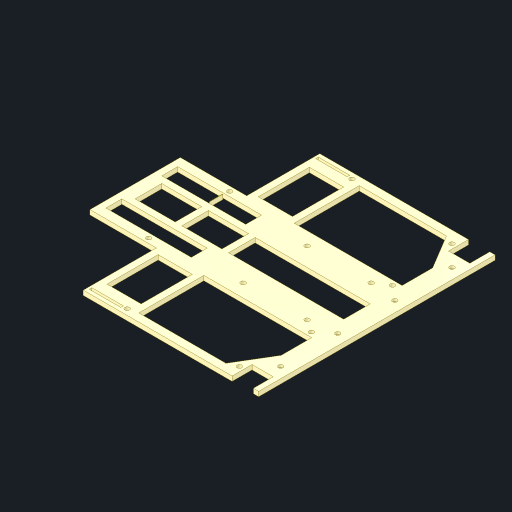
# Autodesk Inventor part: base
Saved by Autodesk Inventor 2023 (Build 270158000, 158)
## iProperties
Created: 2024-04-29
Part Number: base
Material: Nylon 6/6
Document SubType Name: Modeling
Designer: szymo
Density: 1.13 g/cm^3
Appearance: Nylon 6
Mass: 48.7008 g
Surface Area: 329.425 cm^2
Volume: 43.0981 cm^3
Author: szymo
Autodesk Inventor part; units mm, degrees
ref_plane "YZ Plane" through (0, 0, 0) normal (1, 0, 0) x (0, 1, 0)
ref_plane "XZ Plane" through (0, 0, 0) normal (0, 1, 0) x (-1, 0, 0)
ref_plane "XY Plane" through (0, 0, 0) normal (0, 0, 1) x (1, 0, 0)
sketch "Sketch1" plane through (0, 0, 0) normal (0, 1, 0) x (-1, 0, 0)
  line L0 (99, 89) -> (-99, 89)
  line L1 (-99, 89) -> (-99, -89)
  line L2 (-99, -89) -> (99, -89)
  line L3 (99, -89) -> (99, 89)
  line L4 (99, 89) -> (-99, -89) construction
  line L5 (-99, 89) -> (99, -89) construction
  line L6 (-99, 89) -> (-85, 89)
  line L7 (-85, 89) -> (-85, -89)
  line L8 (-85, -89) -> (-99, -89)
  line L9 (-99, -89) -> (-99, 89)
  line L10 (99, 89) -> (97, 89)
  line L11 (97, 89) -> (97, -89)
  line L12 (97, -89) -> (99, -89)
  line L13 (99, -89) -> (99, 89)
  line L14 (97, 33) -> (97, 35)
  line L15 (97, -33) -> (97, -35)
  line L16 (97, 32.8) -> (97, 35)
  line L17 (97, -32.8) -> (97, -35)
  line L18 (97, 89) -> (47, 89)
  line L19 (47, 89) -> (47, 34)
  line L20 (47, 34) -> (97, 34)
  line L21 (97, 34) -> (97, 89)
  line L22 (97, -89) -> (47, -89)
  line L23 (47, -89) -> (47, -34)
  line L24 (47, -34) -> (97, -34)
  line L25 (97, -34) -> (97, -89)
  line L26 (66.5, 33) -> (77.5, 33) projected
  line L27 (77.5, -33) -> (66.5, -33) projected
  line L28 (-81, 74) -> (-81, 89) projected
  line L29 (-81, 31) -> (-81, 55) projected
  line L30 (-81, -12) -> (-81, 12) projected
  line L31 (-81, -55) -> (-81, -31) projected
  line L32 (-81, -89) -> (-81, -74) projected
  arc A0 (-81, 74) -> (-79, 72) centre (-79, 74) ccw projected
  line L33 (-70, 72) -> (-79, 72) projected
  line L34 (-70, 57) -> (-70, 72) projected
  line L35 (-79, 57) -> (-70, 57) projected
  arc A1 (-79, 57) -> (-81, 55) centre (-79, 55) ccw projected
  arc A2 (-81, 31) -> (-79, 29) centre (-79, 31) ccw projected
  line L36 (-70, 29) -> (-79, 29) projected
  line L37 (-70, 14) -> (-70, 29) projected
  line L38 (-79, 14) -> (-70, 14) projected
  arc A3 (-79, 14) -> (-81, 12) centre (-79, 12) ccw projected
  arc A4 (-81, -12) -> (-79, -14) centre (-79, -12) ccw projected
  line L39 (-70, -14) -> (-79, -14) projected
  line L40 (-70, -29) -> (-70, -14) projected
  line L41 (-79, -29) -> (-70, -29) projected
  arc A5 (-79, -29) -> (-81, -31) centre (-79, -31) ccw projected
  arc A6 (-81, -55) -> (-79, -57) centre (-79, -55) ccw projected
  line L42 (-70, -57) -> (-79, -57) projected
  line L43 (-70, -72) -> (-70, -57) projected
  line L44 (-79, -72) -> (-70, -72) projected
  arc A7 (-79, -72) -> (-81, -74) centre (-79, -74) ccw projected
  circle A8 centre (-77, -64.5) radius 1.2295 projected
  circle A9 centre (-77, -21.5) radius 1.2295 projected
  circle A10 centre (-77, 21.5) radius 1.2295 projected
  circle A11 centre (-77, 64.5) radius 1.2295 projected
  line L45 (-65, 89) -> (-79, 89)
  line L46 (-79, 89) -> (-79, 75)
  line L47 (-79, 75) -> (-65, 75)
  line L48 (-65, 75) -> (-65, 89)
  line L49 (-65, 89) -> (-81, 89)
  line L50 (-81, 89) -> (-81, 74)
  line L51 (-81, 74) -> (-65, 74)
  line L52 (-65, 74) -> (-65, 89)
  line L53 (-99, 0) -> (97, 0)
  line L54 (0, 0) -> (-99, 0) construction
  line L55 (-65, -89) -> (-79, -89)
  line L56 (-79, -89) -> (-79, -75)
  line L57 (-79, -75) -> (-65, -75)
  line L58 (-65, -75) -> (-65, -89)
  line L59 (-65, -89) -> (-81, -89)
  line L60 (-81, -89) -> (-81, -74)
  line L61 (-81, -74) -> (-65, -74)
  line L62 (-65, -74) -> (-65, -89)
  point P0 (47, 89)
  point P1 (47, -89)
  point P2 (97, 34)
  point P3 (-81, -89)
  point P4 (-79, -74)
  dimension "d0" = 198
  dimension "d1" = 178
  dimension "d2" = 14
  dimension "d3" = 2
  dimension "d16" = 50
  dimension "d17" = 55
  dimension "d18" = 50
  dimension "d19" = 55
  dimension "d20" = 1
  dimension "d21" = 1
  dimension "d22" = 14
  dimension "d23" = 14
  dimension "d24" = 2
  dimension "d25" = 1
  dimension "d26" = 2
  constraints: 88 end point, 14 parallel, 10 symmetric about line, 8 perpendicular, 8 point on line, 7 horizontal, 4 midpoint, 2 collinear
  measures "d0" distance of L2.end L1.end
  measures "d1" distance of L1.end L0.end
  measures "d2" distance of L7.end L8.end
  measures "d3" distance of L12.end L11.end
  measures "d16" distance of L20.end L19.end
  measures "d17" distance of L19.end L18.end
  measures "d18" distance of L23.end L24.end
  measures "d19" distance of L22.end L23.end
  measures "d20" distance between parallel lines of L20 L26
  measures "d21" distance between parallel lines of L27 L24
  measures "d22" distance of L47.end L46.end
  measures "d23" distance of L46.end L45.end
  measures "d24" distance between parallel lines of L28 L46
  measures "d25" distance between parallel lines of L47 L51
  measures "d26" distance between parallel lines of L33 L51
extrude "Extrusion1" add sketch "Sketch1" along normal blind 3.5 contours L19 L20 L11 L53 L30 A3 L38 L37 L36 A2 L29 A1 L35 L34 L33 A0 L51 L52 L48 L0 | L2 L58 L62 L61 A7 L44 L43 L42 A6 L31 A5 L41 L40 L39 A4 L30 L53 L11 L24 L23 | L28 A0 L33 L34 L35 A1 L29 A2 L36 L37 L38 A3 L30 L53 L7 L0 | L2 L7 L53 L30 A4 L39 L40 L41 A5 L31 A6 L42 L43 L44 A7 L32 | A8 | A9 | A10 | A11
sketch "Sketch3" plane through (0, 0, 0) normal (0, -1, 0) x (1, 0, 0)
  line L0 (65, -74) -> (65, -89) projected
  line L1 (81, -74) -> (65, -74) projected
  line L2 (81, -89) -> (81, -74) projected
  line L3 (85, -89) -> (81, -89) projected
  line L4 (85, 89) -> (85, -89) projected
  line L5 (81, 89) -> (85, 89) projected
  line L6 (81, 74) -> (81, 89) projected
  line L7 (65, 74) -> (81, 74) projected
  line L8 (65, 89) -> (65, 74) projected
  line L9 (-47, 89) -> (65, 89) projected
  line L10 (-47, 34) -> (-47, 89) projected
  line L11 (-97, 34) -> (-47, 34) projected
  line L12 (-97, -34) -> (-97, 34) projected
  line L13 (-47, -34) -> (-97, -34) projected
  line L14 (-47, -89) -> (-47, -34) projected
  line L15 (65, -89) -> (-47, -89) projected
  circle A0 centre (70, 80) radius 1.75 projected
  line L16 (-21.635, 86.2) -> (-21.635, 84.2) projected
  line L17 (-21.635, 84.2) -> (-45.325, 84.2) projected
  line L18 (-45.325, 84.2) -> (-45.325, 86.2) projected
  line L19 (-45.325, 86.2) -> (-21.635, 86.2) projected
  line L20 (73, 77) -> (73, 89) projected
  line L21 (-47, 89) -> (73, 89) projected
  line L22 (-47, 89) -> (-47, 76.2) projected
  line L23 (-14.925, 76.2) -> (-47, 76.2) projected
  line L24 (-14.925, 83) -> (-14.925, 76.2) projected
  line L25 (58, 83) -> (-14.925, 83) projected
  line L26 (58, 77) -> (58, 83) projected
  line L27 (73, 77) -> (58, 77) projected
  circle A1 centre (-18.3706, 84.6) radius 1.8 projected
  circle A2 centre (61.5, 80) radius 1.8 projected
  circle A3 centre (70, -83) radius 1.75 projected
  line L28 (-21.635, -86.2) -> (-21.635, -84.2) projected
  line L29 (-45.325, -86.2) -> (-21.635, -86.2) projected
  line L30 (-45.325, -84.2) -> (-45.325, -86.2) projected
  line L31 (-21.635, -84.2) -> (-45.325, -84.2) projected
  line L32 (73, -77) -> (73, -89) projected
  line L33 (73, -77) -> (58, -77) projected
  line L34 (58, -77) -> (58, -83) projected
  line L35 (58, -83) -> (-14.925, -83) projected
  line L36 (-14.925, -83) -> (-14.925, -76.2) projected
  line L37 (-14.925, -76.2) -> (-47, -76.2) projected
  line L38 (-47, -89) -> (-47, -76.2) projected
  line L39 (-47, -89) -> (73, -89) projected
  circle A4 centre (-18.3706, -84.6) radius 1.8 projected
  circle A5 centre (61.5, -80) radius 1.8 projected
  line L40 (-16.25, -37.7) -> (-47, -37.7) projected
  line L41 (-16.25, -37.7) -> (-16.25, -34.2) projected
  line L42 (-16.25, -34.2) -> (-47, -34.2) projected
  line L43 (-47, -37.7) -> (-47, -34.2) projected
  circle A6 centre (66.25, -30.5) radius 1.8 projected
  circle A7 centre (-56.325, -30.5) radius 1.8 projected
  line L44 (69.5, -34) -> (69.5, -27) projected
  line L45 (69.5, -27) -> (-97, -27) projected
  line L46 (-97, -27) -> (-97, -34) projected
  line L47 (-97, -34) -> (-94, -34) projected
  line L48 (-94, -34) -> (41.0514, -34) projected
  line L49 (41.0514, -34) -> (41.0514, -45) projected
  line L50 (41.0514, -45) -> (45.7494, -45) projected
  line L51 (45.7494, -45) -> (45.7494, -34.8203) projected
  line L52 (45.7494, -45) -> (59.075, -45) projected
  line L53 (59.075, -34) -> (59.075, -45) projected
  line L54 (59.075, -34) -> (69.5, -34) projected
  line L55 (-16.65, -10) -> (-16.65, -27) projected
  line L56 (-16.65, -10) -> (-97, -10) projected
  line L57 (-97, -15) -> (-97, -10) projected
  line L58 (-97, -15) -> (-17.65, -15) projected
  line L59 (-17.65, -15) -> (-17.65, -27) projected
  line L60 (-16.65, -27) -> (-17.65, -27) projected
  line L61 (-16.65, 10) -> (-16.65, 27) projected
  line L62 (-16.65, 27) -> (-17.65, 27) projected
  line L63 (-17.65, 15) -> (-17.65, 27) projected
  line L64 (-97, 15) -> (-17.65, 15) projected
  line L65 (-97, 15) -> (-97, 10) projected
  line L66 (-16.65, 10) -> (-97, 10) projected
  line L67 (-16.25, 37.7) -> (-47, 37.7) projected
  line L68 (-47, 37.7) -> (-47, 34.2) projected
  line L69 (-16.25, 34.2) -> (-47, 34.2) projected
  line L70 (-16.25, 37.7) -> (-16.25, 34.2) projected
  circle A8 centre (66.25, 30.5) radius 1.8 projected
  circle A9 centre (-56.325, 30.5) radius 1.8 projected
  line L71 (69.5, 34) -> (69.5, 27) projected
  line L72 (59.075, 34) -> (69.5, 34) projected
  line L73 (59.075, 34) -> (59.075, 45) projected
  line L74 (45.7494, 45) -> (59.075, 45) projected
  line L75 (45.7494, 45) -> (45.7494, 34.8203) projected
  line L76 (41.0514, 45) -> (45.7494, 45) projected
  line L77 (41.0514, 34) -> (41.0514, 45) projected
  line L78 (-94, 34) -> (41.0514, 34) projected
  line L79 (-97, 34) -> (-94, 34) projected
  line L80 (-97, 27) -> (-97, 34) projected
  line L81 (69.5, 27) -> (-97, 27) projected
  circle A10 centre (77, 21.5) radius 1.2295 projected
  circle A11 centre (77, -64.5) radius 1.2295 projected
  circle A12 centre (77, -21.5) radius 1.2295 projected
  circle A13 centre (77, 64.5) radius 1.2295 projected
  line L82 (70, -72) -> (79, -72) projected
  arc A14 (81, -74) -> (79, -72) centre (79, -74) ccw projected
  line L83 (81, -74) -> (81, -89) projected
  line L84 (81, -89) -> (85, -89) projected
  line L85 (85, -89) -> (85, 89) projected
  line L86 (81, 89) -> (85, 89) projected
  line L87 (81, 89) -> (81, 74) projected
  arc A15 (79, 72) -> (81, 74) centre (79, 74) ccw projected
  line L88 (79, 72) -> (70, 72) projected
  line L89 (70, 57) -> (70, 72) projected
  line L90 (70, 57) -> (79, 57) projected
  arc A16 (81, 55) -> (79, 57) centre (79, 55) ccw projected
  line L91 (81, 55) -> (81, 31) projected
  arc A17 (79, 29) -> (81, 31) centre (79, 31) ccw projected
  line L92 (79, 29) -> (70, 29) projected
  line L93 (70, 14) -> (70, 29) projected
  line L94 (70, 14) -> (79, 14) projected
  arc A18 (81, 12) -> (79, 14) centre (79, 12) ccw projected
  line L95 (81, 12) -> (81, -12) projected
  arc A19 (79, -14) -> (81, -12) centre (79, -12) ccw projected
  line L96 (79, -14) -> (70, -14) projected
  line L97 (70, -29) -> (70, -14) projected
  line L98 (70, -29) -> (79, -29) projected
  arc A20 (81, -31) -> (79, -29) centre (79, -31) ccw projected
  line L99 (81, -31) -> (81, -55) projected
  arc A21 (79, -57) -> (81, -55) centre (79, -55) ccw projected
  line L100 (79, -57) -> (70, -57) projected
  line L101 (70, -72) -> (70, -57) projected
  line L102 (85, 89) -> (70, 89)
  line L103 (70, 89) -> (70, -89)
  line L104 (65, -89) -> (85, -89)
  line L105 (85, -89) -> (85, 89)
  line L106 (85, 34) -> (-97, 34)
  line L107 (-97, 34) -> (-97, 10)
  line L108 (-97, 10) -> (85, 10)
  line L109 (85, 10) -> (85, 34)
  line L110 (-97, -10) -> (85, -10)
  line L111 (85, -10) -> (85, -34)
  line L112 (85, -34) -> (-97, -34)
  line L113 (-97, -34) -> (-97, -10)
  line L114 (-47, 34) -> (-47, 34.2)
  line L115 (-47, 34.2) -> (-97, 34)
  line L116 (-97, -34) -> (-47, -34.2)
  line L117 (-47, -34.2) -> (-47, -34)
  line L118 (70, 89) -> (58, 89)
  line L119 (58, 89) -> (58, 77)
  line L120 (58, 77) -> (70, 77)
  line L121 (70, 77) -> (70, 89)
  line L122 (58, 89) -> (-14.925, 89)
  line L123 (-14.925, 89) -> (-14.925, 83)
  line L124 (-14.925, 83) -> (58, 83)
  line L125 (58, 83) -> (58, 89)
  line L126 (-14.925, 89) -> (-47, 89)
  line L127 (-47, 89) -> (-47, 76.2)
  line L128 (-47, 76.2) -> (-14.925, 76.2)
  line L129 (-14.925, 76.2) -> (-14.925, 89)
  line L130 (65, -77) -> (58, -77)
  line L131 (58, -77) -> (58, -89)
  line L132 (58, -89) -> (70, -89)
  line L133 (70, -89) -> (70, -77)
  line L134 (58, -89) -> (-14.925, -89)
  line L135 (-14.925, -89) -> (-14.925, -83)
  line L136 (-14.925, -83) -> (58, -83)
  line L137 (58, -83) -> (58, -89)
  line L138 (-14.925, -89) -> (-47, -89)
  line L139 (-47, -89) -> (-47, -76.2)
  line L140 (-47, -76.2) -> (-14.925, -76.2)
  line L141 (-14.925, -76.2) -> (-14.925, -89)
  line L142 (-47, -76.2) -> (-42, -76.2)
  line L143 (-42, -76.2) -> (-42, -34)
  line L144 (-42, -34) -> (-47, -34)
  line L145 (-47, -34) -> (-47, -76.2)
  line L146 (-47, 76.2) -> (-42, 76.2)
  line L147 (-42, 76.2) -> (-42, 34)
  line L148 (-42, 34) -> (-47, 34)
  line L149 (-47, 34) -> (-47, 76.2)
  line L150 (-16.25, 34.2) -> (-11.25, 34.2)
  line L151 (-11.25, 34.2) -> (-11.25, 83)
  line L152 (-11.25, 83) -> (-16.25, 83)
  line L153 (-16.25, 83) -> (-16.25, 34.2)
  line L154 (-16.25, -34.2) -> (-11.25, -34.2)
  line L155 (-11.25, -34.2) -> (-11.25, -83)
  line L156 (-11.25, -83) -> (-16.25, -83)
  line L157 (-16.25, -83) -> (-16.25, -34.2)
  line L158 (-16.65, 10) -> (-21.65, 10)
  line L159 (-21.65, 10) -> (-21.65, -10)
  line L160 (-21.65, -10) -> (-16.65, -10)
  line L161 (-16.65, -10) -> (-16.65, 10)
  line L162 (-97, 10) -> (-87, 10)
  line L163 (-87, 10) -> (-87, -10)
  line L164 (-87, -10) -> (-97, -10)
  line L165 (-97, -10) -> (-97, 10)
  line L166 (-51.825, 10) -> (-56.825, 10)
  line L167 (-56.825, 10) -> (-56.825, -10)
  line L168 (-56.825, -10) -> (-51.825, -10)
  line L169 (-51.825, -10) -> (-51.825, 10)
  line L170 (-16.25, 34.2) -> (-16.25, 34)
  line L171 (-11.25, 34.2) -> (-11.25, 34)
  line L172 (-11.25, -34.2) -> (-11.25, -34)
  line L173 (-16.25, -34.2) -> (-16.25, -34)
  line L174 (70, 57) -> (54.4, 83)
  line L175 (70, -57) -> (54.4, -83)
  line L176 (-34.0117, 16) -> (-34.0117, 26)
  line L177 (-34.0117, 26) -> (-32.704, 26)
  line L178 (-32.704, 26) -> (-32.704, 16)
  line L179 (-32.704, 16) -> (-34.0117, 16)
  line L180 (-35.6343, 26) -> (-35.6343, 16)
  line L181 (-35.6343, 16) -> (-50.4468, 16)
  line L182 (-50.4468, 16) -> (-50.4468, 26)
  line L183 (-50.4468, 26) -> (-35.6343, 26)
  line L184 (-66.4245, 19) -> (-72.4408, 19)
  line L185 (-72.4408, 19) -> (-72.4408, 23)
  line L186 (-72.4408, 23) -> (-66.4245, 23)
  line L187 (-66.4245, 23) -> (-66.4245, 19)
  line L188 (-82.583, 26) -> (-82.583, 23)
  line L189 (-82.583, 23) -> (-80.9671, 23)
  line L190 (-80.9671, 23) -> (-80.9671, 19)
  line L191 (-80.9671, 19) -> (-82.583, 19)
  line L192 (-82.583, 19) -> (-82.583, 16)
  line L193 (-82.583, 16) -> (-86.007, 16)
  spline S0 degree 3 poles (-86.007, 16) (-86.007, 17.6667) (-86.007, 19.3333) (-86.007, 22.6667) (-86.007, 24.3333) (-86.007, 26) knots -1 -1 -1 -1 -0.5 -0.5 0 0 0 0
  line L194 (-86.007, 26) -> (-82.583, 26)
  line L195 (-61.417, 23) -> (-61.417, 26)
  line L196 (-61.417, 26) -> (-57.3554, 26)
  spline S1 degree 3 poles (-57.3554, 26) (-57.3554, 24.3333) (-57.3554, 22.6667) (-57.3554, 19.3333) (-57.3554, 17.6667) (-57.3554, 16) knots -1 -1 -1 -1 -0.5 -0.5 0 0 0 0
  line L197 (-57.3554, 16) -> (-61.417, 16)
  line L198 (-61.417, 16) -> (-61.417, 19)
  line L199 (-61.417, 19) -> (-62.6269, 19)
  line L200 (-62.6269, 19) -> (-62.6269, 23)
  line L201 (-62.6269, 23) -> (-61.417, 23)
  line L202 (-57.2691, 26) -> (-57.2691, 16)
  line L203 (-86.7309, 16) -> (-86.7309, 26)
  line L204 (-49.6101, -16) -> (-49.6101, -26)
  line L205 (-49.6101, -26) -> (-51.9631, -26)
  line L206 (-51.9631, -26) -> (-51.9631, -16)
  line L207 (-51.9631, -16) -> (-49.6101, -16)
  line L208 (-33.7735, -16) -> (-33.7735, -26)
  line L209 (-33.7735, -26) -> (-49.1385, -26)
  line L210 (-49.1385, -26) -> (-49.1385, -16)
  line L211 (-49.1385, -16) -> (-33.7735, -16)
  line L212 (-61.417, -26) -> (-61.417, -23)
  line L213 (-61.417, -23) -> (-69.2128, -23)
  line L214 (-69.2128, -23) -> (-69.2128, -19)
  line L215 (-69.2128, -19) -> (-61.417, -19)
  line L216 (-61.417, -19) -> (-61.417, -16)
  line L217 (-61.417, -16) -> (-57.0283, -16)
  spline S2 degree 3 poles (-57.0283, -16) (-57.0283, -17.6667) (-57.0283, -19.3333) (-57.0283, -22.6667) (-57.0283, -24.3333) (-57.0283, -26) knots -1 -1 -1 -1 -0.5 -0.5 0 0 0 0
  line L218 (-57.0283, -26) -> (-61.417, -26)
  line L219 (-82.583, -23) -> (-82.583, -26)
  line L220 (-82.583, -26) -> (-85.6557, -26)
  spline S3 degree 3 poles (-85.6557, -26) (-85.6557, -24.3333) (-85.6557, -22.6667) (-85.6557, -19.3333) (-85.6557, -17.6667) (-85.6557, -16) knots -1 -1 -1 -1 -0.5 -0.5 0 0 0 0
  line L221 (-85.6557, -16) -> (-82.583, -16)
  line L222 (-82.583, -16) -> (-82.583, -19)
  line L223 (-82.583, -19) -> (-78.6331, -19)
  line L224 (-78.6331, -19) -> (-78.6331, -23)
  line L225 (-78.6331, -23) -> (-82.583, -23)
  line L226 (-57.2691, -16) -> (-57.2691, -26)
  line L227 (-86.7309, -26) -> (-86.7309, -16)
  line L228 (-27.704, 27) -> (-27.704, 15)
  line L229 (-92, 15) -> (-92, 27)
  line L230 (-92, -15) -> (-92, -27)
  line L231 (-28.7735, -15) -> (-28.7735, -27)
  point P0 (0, 0)
  point P1 (-16.25, -76.2)
  point P2 (-42, -37.7)
  point P3 (-16.25, 76.2)
  point P4 (-42, 37.7)
  point P5 (-87, -10)
  point P6 (70, -10)
  point P7 (70, 10)
  point P8 (70, -34)
  point P9 (70, 34)
  dimension "d27" = 5
  dimension "d28" = 5
  dimension "d29" = 5
  dimension "d30" = 5
  dimension "d31" = 5
  dimension "d32" = 10
  dimension "d33" = 5
  dimension "d34" = 30.175
  dimension "d35" = 30.175
  dimension "d36" = 15
  dimension "d37" = 0
  dimension "d38" = 0
  dimension "d41" = 5
  dimension "d42" = 5
  dimension "d43" = 5.2691
  dimension "d44" = 5.2691
  dimension "d45" = 5
  dimension "d46" = 5
  constraints: 260 end point, 42 horizontal, 32 parallel, 29 point on line, 26 vertical, 24 perpendicular, 4 collinear, 4 vertical alignment, 68 other
  measures "d27" distance of L144.end L143.end
  measures "d28" distance of L147.end L148.end
  measures "d29" distance of L152.end L151.end
  measures "d30" distance of L155.end L156.end
  measures "d31" distance of L160.end L159.end
  measures "d32" distance of L163.end L164.end
  measures "d33" distance of L168.end L167.end
  measures "d34" distance between parallel lines of L159 L169
  measures "d35" distance between parallel lines of L167 L163
  measures "d36" distance between parallel lines of L4 L103
  measures "d37" distance from line of L174 L26.start
  measures "d38" distance from line of L175 L33.end
  measures "d41" distance between parallel lines of L228 L178
  measures "d42" distance between parallel lines of L231 L208
  measures "d43" distance between parallel lines of L230 L227
  measures "d44" distance between parallel lines of L203 L229
  measures "d45" distance between parallel lines of L229 L107
  measures "d46" distance between parallel lines of L230 L12
extrude "Extrusion2" cut sketch "Sketch3" against normal blind 10 contours L175 L35 L155 L172 L48 L49 L50 L52 L53 L54 L112 L103 | L53 L52 L50 L49 L112 | L143 L40 L157 L37 | L110 L161 L108 L103 | L56 L169 L66 L159 | L45 L230 L58 L231 | L106 L72 L73 L74 L76 L77 L78 L171 L151 L25 L174 L103 | L56 L163 L66 L167 | L228 L64 L229 L81 | L106 L77 L76 L74 L73 | L153 L67 L147 L23 | L16 L17 L18 L19 | L29 L30 L31 L28 | L176 L177 L178 L179 | L180 L181 L182 L183 | L184 L185 L186 L187 | L188 L189 L190 L191 L192 L193 S0 L194 | L195 L196 S1 L197 L198 L199 L200 L201 | L204 L205 L206 L207 | L208 L209 L210 L211 | L212 L213 L214 L215 L216 L217 L226 L218 | L219 L220 S3 L221 L222 L223 L224 L225
sketch "Sketch4" plane through (0, 0, 0) normal (0, -1, 0) x (1, 0, 0)
  circle A0 centre (-56.325, 30.5) radius 3 projected
  circle A1 centre (-56.325, -30.5) radius 3 projected
  circle A2 centre (66.25, 30.5) radius 1.8 projected
  circle A3 centre (66.25, -30.5) radius 1.8 projected
  circle A4 centre (61.5, -80) radius 1.8 projected
  circle A5 centre (61.5, 80) radius 1.8 projected
  circle A6 centre (-18.3706, 84.6) radius 1.8 projected
  circle A7 centre (-18.3706, -84.6) radius 1.8 projected
  circle A8 centre (8.4, 24.1) radius 1.6 projected
  circle A9 centre (8.4, -24.1) radius 1.6 projected
  circle A10 centre (56.6, -24.1) radius 1.6 projected
  circle A11 centre (56.6, 24.1) radius 1.6 projected
  point P0 (0, 0)
  constraints: 12 coincident
hole "Hole1" at (-56.325, 0, -30.5) at (-56.325, 0, 30.5) at (-18.3706, 0, 84.6) at (-18.3706, 0, -84.6) at (8.4, 0, -24.1) at (8.4, 0, 24.1) at (56.6, 0, 24.1) at (61.5, 0, 80) at (66.25, 0, 30.5) at (56.6, 0, -24.1) at (66.25, 0, -30.5) at (61.5, 0, -80) direction (0, 1, 0) diameter 3.6 end through all counterbore diameter 11 counterbore depth 0 clearance for "Hex Head Cap Screw ISO 24014 (Spotface)" size "M3" standard "ISO"
sketch "Sketch5" plane through (0, 0, 0) normal (0, -1, 0) x (1, 0, 0)
  circle A0 centre (77, 21.5) radius 1.2295 projected
  circle A1 centre (77, -64.5) radius 1.2295 projected
  circle A2 centre (77, -21.5) radius 1.2295 projected
  circle A3 centre (77, 64.5) radius 1.2295 projected
  line L0 (79, -72) -> (70, -72) projected
  line L1 (70, -72) -> (70, -57) projected
  line L2 (70, -57) -> (79, -57) projected
  arc A4 (79, -57) -> (81, -55) centre (79, -55) ccw projected
  line L3 (81, -55) -> (81, -31) projected
  arc A5 (81, -31) -> (79, -29) centre (79, -31) ccw projected
  line L4 (79, -29) -> (70, -29) projected
  line L5 (70, -29) -> (70, -14) projected
  line L6 (70, -14) -> (79, -14) projected
  arc A6 (79, -14) -> (81, -12) centre (79, -12) ccw projected
  line L7 (81, -12) -> (81, 12) projected
  arc A7 (81, 12) -> (79, 14) centre (79, 12) ccw projected
  line L8 (79, 14) -> (70, 14) projected
  line L9 (70, 14) -> (70, 29) projected
  line L10 (70, 29) -> (79, 29) projected
  arc A8 (79, 29) -> (81, 31) centre (79, 31) ccw projected
  line L11 (81, 31) -> (81, 55) projected
  arc A9 (81, 55) -> (79, 57) centre (79, 55) ccw projected
  line L12 (79, 57) -> (70, 57) projected
  line L13 (70, 57) -> (70, 72) projected
  line L14 (70, 72) -> (79, 72) projected
  arc A10 (79, 72) -> (81, 74) centre (79, 74) ccw projected
  line L15 (81, 74) -> (81, 89) projected
  line L16 (85, 89) -> (81, 89) projected
  line L17 (85, -89) -> (85, 89) projected
  line L18 (85, -89) -> (81, -89) projected
  line L19 (81, -89) -> (81, -74) projected
  arc A11 (81, -74) -> (79, -72) centre (79, -74) ccw projected
  point P0 (0, 0)
  constraints: 4 coincident
hole "Hole2" at (77, 0, -64.5) at (77, 0, -21.5) at (77, 0, 21.5) at (77, 0, 64.5) direction (0, 1, 0) diameter 3.6 end through all countersink diameter 6.7 countersink angle 90
equation "\"d34\" = d35"
body "Solid1"
